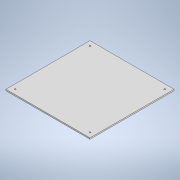
# Autodesk Inventor part: lid_bakeout_box_2020_iqc
Saved by Autodesk Inventor 2020.2 (Build 242310000, 310)
## iProperties
Created: 2020-01-23
Part Number: lid_bakeout_box_2020_iqc
Material: Generic
Document SubType Name: Modeling
Designer: ColinP
Density: 1 g/cm^3
Appearance: Default
Author: ColinP
Autodesk Inventor part; units mm, degrees
ref_plane "YZ Plane" through (0, 0, 0) normal (1, 0, 0) x (0, 1, 0)
ref_plane "XZ Plane" through (0, 0, 0) normal (0, 1, 0) x (-1, 0, 0)
ref_plane "XY Plane" through (0, 0, 0) normal (0, 0, 1) x (1, 0, 0)
sketch "Sketch1" plane through (0, 0, 0) normal (0, 1, 0) x (-1, 0, 0)
  line L0 (254, 254) -> (0, 254)
  line L1 (0, 254) -> (0, 0)
  line L2 (0, 0) -> (254, 0)
  line L3 (254, 0) -> (254, 254)
  constraints: 8 end point, 2 parallel, 1 horizontal, 1 perpendicular
extrude "Extrusion1" add sketch "Sketch1" along normal blind 4
sketch "Sketch2" plane through (0, 4, 0) normal (0, 1, 0) x (1, 0, 0)
  line L0 (-254, -254) -> (0, -254) projected
  line L1 (0, -254) -> (0, -240)
  line L2 (0, -254) -> (0, 0) projected
  line L3 (0, -240) -> (-14, -240)
  line L4 (-14, -240) -> (-14, -14)
  line L5 (-14, -14) -> (-240, -14)
  line L6 (-240, -14) -> (-240, -240)
  dimension "d2" = 14
  dimension "d3" = 14
  dimension "d4" = 226
  dimension "d5" = 226
  dimension "d6" = 226
  constraints: 10 end point, 3 perpendicular, 2 point on line
  measures "d2" distance of L0.end L1.end
  measures "d3" distance of L1.end L3.end
  measures "d4" distance of L3.end L4.end
  measures "d5" distance of L4.end L5.end
  measures "d6" distance of L5.end L6.end
hole "Hole1" at (-14, 4, 14) at (-14, 4, 240) at (-240, 4, 14) at (-240, 4, 240) direction (0, -1, 0) diameter 4.1148 depth 12.3
body "Solid1"
